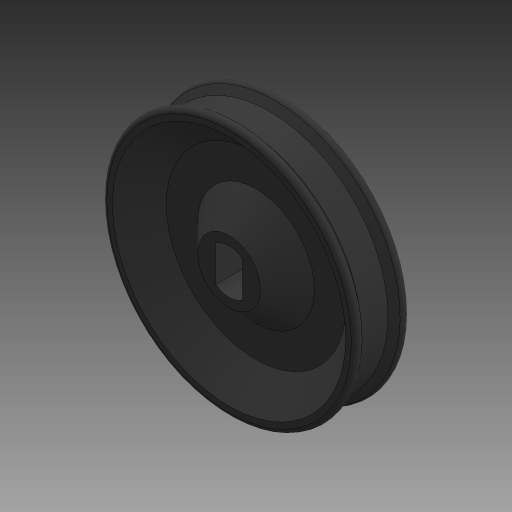
# Autodesk Inventor part: rub-ring
Saved by Autodesk Inventor 2023 (Build 270158000, 158)
## iProperties
Created: 2024-02-02
Part Number: rub-ring
Material: Všeobecné
Document SubType Name: Modeling
Designer: matej
Mass: 2.35927 g
Surface Area: 19.8158 cm^2
Volume: 2.35927 cm^3
Density: 1 g/cm^3
Appearance: Guma – černá
Author: matej
## iProperties of the stored document rub-ring_3D tisk.ipt
Created: 2024-02-02
Part Number: rub-ring_3D tisk
Material: Všeobecné
Document SubType Name: Modeling
Designer: matej
Mass: 2.35927 g
Surface Area: 19.8158 cm^2
Volume: 2.35927 cm^3
Density: 1 g/cm^3
Appearance: Výchozí
Author: matej
Autodesk Inventor part; units mm, degrees
ref_plane "YZ Plane" through (0, 0, 0) normal (1, 0, 0) x (0, 1, 0)
ref_plane "XZ Plane" through (0, 0, 0) normal (0, 1, 0) x (-1, 0, 0)
ref_plane "XY Plane" through (0, 0, 0) normal (0, 0, 1) x (1, 0, 0)
sketch "Náčrt1" plane through (0, 0, 0) normal (0, 0, 1) x (1, 0, 0)
  circle A0 centre (0, 0) radius 2.5
  line L0 (-1.5, -2.5) -> (1.5, -2.5)
  line L1 (1.5, -2.5) -> (1.5, 2.5)
  line L2 (1.5, 2.5) -> (-1.5, 2.5)
  line L3 (-1.5, 2.5) -> (-1.5, -2.5)
  line L4 (-1.5, -2.5) -> (1.5, 2.5) construction
  line L5 (1.5, -2.5) -> (-1.5, 2.5) construction
  circle A1 centre (0, 0) radius 15
  point P0 (-1.5, -2)
  point P1 (-1.5, 2)
  point P2 (1.5, 2)
  point P3 (1.5, -2)
  dimension "d0" = 5
  dimension "d1" = 3
  dimension "d2" = 5
  dimension "d3" = 30
  constraints: 12 end point, 2 centre point, 2 coincident, 2 midpoint, 2 parallel, 1 horizontal, 1 perpendicular
  measures "d0" diameter of A0
  measures "d1" distance of L2.end L1.end
  measures "d2" distance of L1.end L0.end
  measures "d3" diameter of A1
extrude "Vysunutí1" add sketch "Náčrt1" along normal mid plane 6 contours A0 L1 | A0 L2 L1 | L1 L0 A0 | A0 L3 L2 | L0 L3 A0 | L3 A0 | A1
sketch "Náčrt2" plane through (0, 0, 0) normal (1, 0, 0) x (0, 1, 0)
  line L0 (-15, -3) -> (15, -3) projected
  line L1 (15, 3) -> (15, -3)
  line L2 (15, -3) -> (13.2124, -1.5)
  line L3 (15, -3) -> (17.3336, -3) construction
  line L4 (15, 3) -> (-15, 3) projected
  line L5 (15, 3) -> (13.2124, 1.5)
  line L6 (15, 3) -> (17.3336, 3) construction
  line L7 (13.2124, 1.5) -> (13.2124, -1.5)
  line L8 (0, -7) -> (0, 7) projected
  point P0 (0, 0)
  dimension "d15" = 140
  dimension "d16" = 140
  dimension "d18" = 3
  dimension "d27" = 13.2124
  dimension "d28" = 1.5
  constraints: 12 end point, 2 equal length, 2 horizontal, 1 perpendicular, 1 vertical, 1 other
  measures "d15" angle of L3 L2
  measures "d16" angle of L5 L6
  measures "d18" distance of L5.end L2.end
  measures "d27" distance between parallel lines of L7 L8
revolve "Rotace1" cut sketch "Náčrt2" angle 360 about axis through (0, 0, -10) along (0, 0, 1) contours L2 L7 L5 L1
fillet "Zaoblení1" radius 0.5 2 edges at (0, -15, -3) (0, -15, 3)
sketch "Náčrt3" plane through (0, 0, 3) normal (0, 0, 1) x (1, 0, 0)
  circle A0 centre (0, 0) radius 3.5
  circle A1 centre (0, 0) radius 10
  dimension "d12" = 7
  dimension "d13" = 20
  constraints: 2 centre point, 2 coincident
  measures "d12" diameter of A0
  measures "d13" diameter of A1
extrude "Vysunutí2" cut sketch "Náčrt3" against normal blind 3
chamfer "Zkosení1" distance 3 angle 45 1 edges at (-10, 0, 3)
chamfer "Zkosení2" distance 3 angle 45 1 edges at (-3.5, 0, 0)
equation "\"d15\" = d16"
